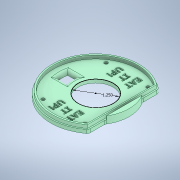
# Autodesk Inventor part: camHolderTop
Saved by Autodesk Inventor 2020 (Build 240168000, 168)
## iProperties
Created: 2020-02-08
Part Number: camHolderTop
Material: Generic
Document SubType Name: Modeling
Designer: Chris Gerth
Density: 1 g/cm^3
Appearance: Default(1)
Author: Chris Gerth
Autodesk Inventor part; units mm, degrees
ref_plane "YZ Plane" through (0, 0, 0) normal (1, 0, 0) x (0, 1, 0)
ref_plane "XZ Plane" through (0, 0, 0) normal (0, 1, 0) x (-1, 0, 0)
ref_plane "XY Plane" through (0, 0, 0) normal (0, 0, 1) x (1, 0, 0)
sketch "Sketch1" plane through (0, 0, 0) normal (0, 1, 0) x (-1, 0, 0)
  arc A0 (-25.4, -31.7246) -> (-25.4, 31.7246) centre (0, 0) ccw
  line L0 (-25.4, 31.7246) -> (-25.4, -31.7246)
  dimension "d0" = 81.28
  dimension "d21" = 25.4
  constraints: 2 end point, 2 point on circle, 1 centre point, 1 coincident, 1 vertical
  measures "d0" diameter of A0
  measures "d21" distance from line of L0 point (0, 0)
extrude "Extrusion1" add sketch "Sketch1" along normal blind 3.175
sketch "Sketch2" plane through (0, 3.175, 0) normal (0, 1, 0) x (0, 0, 1)
  circle A0 centre (0, 0) radius 40.64
  arc A1 (-31.3667, 24.003) -> (31.3667, 24.003) centre (0, 0) ccw
  arc A2 (-31.7246, 25.4) -> (31.7246, 25.4) centre (0, 0) ccw projected
  line L0 (31.7246, 25.4) -> (-31.7246, 25.4)
  line L1 (31.3667, 24.003) -> (-31.3667, 24.003)
  line L2 (30.48, 22.86) -> (-30.48, 22.86)
  arc A3 (-30.48, 22.86) -> (30.48, 22.86) centre (0, 0) ccw
  dimension "d3" = 81.28
  dimension "d5" = 78.994
  dimension "d22" = 1.397
  dimension "d23" = 1.143
  constraints: 6 end point, 4 point on circle, 3 centre point, 3 coincident, 3 horizontal
  measures "d3" diameter of A0
  measures "d5" diameter of A1
  measures "d22" distance between parallel lines of L1 L0
  measures "d23" distance between parallel lines of L1 L2
extrude "Extrusion2" add sketch "Sketch2" along normal blind 3.048 contours L1 A1
sketch "Sketch3" plane through (0, 3.175, 0) normal (0, 1, 0) x (0, 0, 1)
  circle A0 centre (0, 0) radius 15.875
  dimension "d8" = 31.75
  constraints: 1 centre point, 1 coincident
  measures "d8" diameter of A0
extrude "Extrusion3" cut sketch "Sketch3" against normal up to surface (3.175 mm away)
sketch "Sketch4" plane through (0, 3.175, 0) normal (0, 1, 0) x (0, 0, 1)
  line L0 (28.575, 19.05) -> (28.575, -19.05)
  line L1 (28.575, -19.05) -> (-28.575, -19.05)
  line L2 (-28.575, -19.05) -> (-28.575, 19.05)
  line L3 (-28.575, 19.05) -> (28.575, 19.05)
  line L4 (28.575, 19.05) -> (-28.575, -19.05) construction
  line L5 (28.575, -19.05) -> (-28.575, 19.05) construction
  circle A0 centre (-28.575, -19.05) radius 1.55
  circle A1 centre (-28.575, 19.05) radius 1.55
  circle A2 centre (28.575, 19.05) radius 1.55
  circle A3 centre (28.575, -19.05) radius 1.55
  point P0 (0, 0)
  dimension "d12" = 38.1
  dimension "d13" = 3.1
  dimension "d14" = 3.1
  dimension "d15" = 3.1
  dimension "d16" = 3.1
  dimension "d17" = 57.15
  constraints: 12 end point, 4 centre point, 4 coincident, 2 parallel, 1 perpendicular
  measures "d12" distance of L1.end L2.end
  measures "d13" diameter of A0
  measures "d14" diameter of A1
  measures "d15" diameter of A2
  measures "d16" diameter of A3
  measures "d17" distance of L0.end L1.end
extrude "Extrusion4" cut sketch "Sketch4" against normal up to surface (3.175 mm away) contours L3 A2 L0 | L0 A2 L3 | A3 L1 L0 | L0 L1 A3 | A1 L2 L3 | L3 L2 A1 | A0 L2 L1 | L1 L2 A0
sketch "Sketch5" plane through (0, 3.175, 0) normal (0, 1, 0) x (1, 0, 0)
  circle A0 centre (0, 0) radius 30.48
  line L0 (25.4, -31.7246) -> (25.4, 31.7246) projected
  line L1 (25.4, -16.8485) -> (25.4, 16.8485)
  dimension "d24" = 60.96
  constraints: 2 end point, 2 point on circle, 2 point on line, 1 centre point, 1 coincident
  measures "d24" diameter of A0
extrude "Extrusion5" add sketch "Sketch5" against normal up to surface (3.175 mm away) contours A0 L0 picked at (26.3286, -3.867)
sketch "Sketch6" plane through (0, 3.175, 0) normal (0, 1, 0) x (1, 0, 0)
  circle A0 centre (0, 0) radius 30.48
  arc A1 (25.4, -16.8485) -> (25.4, 16.8485) centre (0, 0) ccw projected
  line L0 (25.781, 16.2595) -> (25.781, -16.2595)
  line L1 (24.003, -31.3667) -> (24.003, 31.3667) projected
  point P0 (25.781, 16.2595)
  dimension "d27" = 1.778
  constraints: 2 end point, 2 point on circle, 1 centre point, 1 coincident, 1 vertical
  measures "d27" distance between parallel lines of L0 L1
extrude "Extrusion6" add sketch "Sketch6" along normal blind 3.175 contours A0 L0
fillet "Fillet1" radius 3.175 4 edges at (25.4, 1.5875, 31.7246) (25.4, 1.5875, -31.7246) (25.4, 1.5875, 16.8485) (25.4, 1.5875, -16.8485)
sketch "Sketch7" plane through (0, 3.175, 0) normal (0, 1, 0) x (1, 0, 0)
  circle A0 centre (0, 0) radius 30.2768
  circle A1 centre (0, 0) radius 22.352
  line L0 (-21.8722, -4.6064) -> (-29.9243, -4.6064)
  line L1 (-21.8866, 4.5376) -> (-29.9348, 4.5376)
  dimension "d31" = 60.5536
  dimension "d32" = 44.704
  dimension "d33" = 9.144
  constraints: 4 end point, 4 point on circle, 2 centre point, 2 coincident, 1 horizontal
  measures "d31" diameter of A0
  measures "d32" diameter of A1
  measures "d33" distance between parallel lines of L1 L0
extrude "Extrusion7" cut sketch "Sketch7" against normal up to surface (3.175 mm away) contours L1 A1 L0 A0 picked at (-24.6978, -3.5938)
fillet "Fillet2" radius 3.175 4 edges at (-22.352, 3.175, 0.0351) (-25.8983, 3.175, 4.6064) (-25.9107, 3.175, -4.5376) (-30.2768, 3.175, 0.0348)
sketch "Sketch8" plane through (0, 3.175, 0) normal (0, 1, 0) x (1, 0, 0)
  line L0 (11.4987, 33.3187) -> (11.2662, 17.0795) construction
  line L1 (11.2662, 17.0795) -> (-1.4145, 17.261) construction
  line L2 (-1.4145, 17.261) -> (-1.1821, 33.5002) construction
  line L3 (-1.1821, 33.5002) -> (11.4987, 33.3187) construction
  line L4 (11.0156, -18.9279) -> (10.7832, -35.1671) construction
  line L5 (10.7832, -35.1671) -> (-1.8976, -34.9856) construction
  line L6 (-1.8976, -34.9856) -> (-1.6651, -18.7464) construction
  line L7 (-1.6651, -18.7464) -> (11.0156, -18.9279) construction
  line L8 (6.3911, 31.4257) -> (11.4705, 31.353)
  line L9 (11.4705, 31.353) -> (11.4214, 27.92)
  line L10 (11.4214, 27.92) -> (10.4541, 27.9338)
  line L11 (10.4541, 27.9338) -> (10.4851, 30.099)
  line L12 (10.4851, 30.099) -> (9.5918, 30.1118)
  line L13 (9.5918, 30.1118) -> (9.5633, 28.1154)
  line L14 (9.5633, 28.1154) -> (8.5959, 28.1292)
  line L15 (8.5959, 28.1292) -> (8.6245, 30.1256)
  line L16 (8.6245, 30.1256) -> (7.3402, 30.144)
  line L17 (7.3402, 30.144) -> (7.3092, 27.9788)
  line L18 (7.3092, 27.9788) -> (6.3419, 27.9927)
  line L19 (6.3419, 27.9927) -> (6.3911, 31.4257)
  line L20 (6.3374, 27.6757) -> (11.3923, 25.8865)
  line L21 (11.3923, 25.8865) -> (11.3724, 24.4952)
  line L22 (11.3724, 24.4952) -> (6.2683, 22.8515)
  line L23 (6.2683, 22.8515) -> (6.2871, 24.1645)
  line L24 (6.2871, 24.1645) -> (7.329, 24.4667)
  line L25 (7.329, 24.4667) -> (7.3518, 26.0638)
  line L26 (7.3518, 26.0638) -> (6.3191, 26.3997)
  line L27 (6.3191, 26.3997) -> (6.3374, 27.6757)
  line L28 (8.255, 24.7334) -> (9.9419, 25.228)
  line L29 (9.9419, 25.228) -> (8.2699, 25.7748)
  line L30 (8.2699, 25.7748) -> (8.255, 24.7334)
  line L31 (6.2471, 21.3696) -> (10.3593, 21.3107)
  line L32 (10.3593, 21.3107) -> (10.3808, 22.8132)
  line L33 (10.3808, 22.8132) -> (11.3481, 22.7993)
  line L34 (11.3481, 22.7993) -> (11.2868, 18.5184)
  line L35 (11.2868, 18.5184) -> (10.3195, 18.5323)
  line L36 (10.3195, 18.5323) -> (10.341, 20.0347)
  line L37 (10.341, 20.0347) -> (6.2289, 20.0936)
  line L38 (6.2289, 20.0936) -> (6.2471, 21.3696)
  line L39 (-2.0492, 26.1654) -> (-2.0101, 28.8986)
  line L40 (-2.0101, 28.8986) -> (-1.1251, 28.8859)
  line L41 (-1.1251, 28.8859) -> (-1.1355, 28.1573)
  line L42 (-1.1355, 28.1573) -> (2.174, 28.11)
  line L43 (2.174, 28.11) -> (2.1844, 28.8386)
  line L44 (2.1844, 28.8386) -> (3.0694, 28.8259)
  line L45 (3.0694, 28.8259) -> (3.0303, 26.0927)
  line L46 (3.0303, 26.0927) -> (2.1453, 26.1053)
  line L47 (2.1453, 26.1053) -> (2.1557, 26.8339)
  line L48 (2.1557, 26.8339) -> (-1.1537, 26.8813)
  line L49 (-1.1537, 26.8813) -> (-1.1642, 26.1527)
  line L50 (-1.1642, 26.1527) -> (-2.0492, 26.1654)
  line L51 (-2.0753, 24.3419) -> (2.0369, 24.283)
  line L52 (2.0369, 24.283) -> (2.0584, 25.7855)
  line L53 (2.0584, 25.7855) -> (3.0257, 25.7716)
  line L54 (3.0257, 25.7716) -> (2.9644, 21.4907)
  line L55 (2.9644, 21.4907) -> (1.9971, 21.5045)
  line L56 (1.9971, 21.5045) -> (2.0186, 23.007)
  line L57 (2.0186, 23.007) -> (-2.0935, 23.0658)
  line L58 (-2.0935, 23.0658) -> (-2.0753, 24.3419)
  spline S0 degree 2 poles (-10.4805, 29.0054) (-10.4658, 30.0304) (-9.4621, 31.1194) (-8.5072, 31.1057) knots 0 0 0 1 2 2 2
  line L59 (-8.5072, 31.1057) -> (-5.2636, 31.0593)
  line L60 (-5.2636, 31.0593) -> (-5.2818, 29.7832)
  line L61 (-5.2818, 29.7832) -> (-8.4513, 29.8286)
  spline S1 degree 2 poles (-8.4513, 29.8286) (-8.9823, 29.8362) (-9.5067, 29.4444) (-9.5132, 28.9916) knots 0 0 0 1 2 2 2
  spline S2 degree 2 poles (-9.5132, 28.9916) (-9.5195, 28.5511) (-9.0273, 28.1324) (-8.4757, 28.1245) knots 0 0 0 1 2 2 2
  line L62 (-8.4757, 28.1245) -> (-5.3062, 28.0791)
  line L63 (-5.3062, 28.0791) -> (-5.3245, 26.8031)
  line L64 (-5.3245, 26.8031) -> (-8.564, 26.8494)
  spline S3 degree 2 poles (-8.564, 26.8494) (-9.5025, 26.8629) (-10.4956, 27.9516) (-10.4805, 29.0054) knots 0 0 0 1 2 2 2
  spline S4 degree 2 poles (-6.9956, 21.94) (-7.3496, 21.945) (-7.9885, 22.1806) (-8.1996, 22.3936) knots 0 0 0 1 2 2 2
  spline S5 degree 2 poles (-8.1996, 22.3936) (-8.3336, 22.5232) (-8.5514, 22.8392) (-8.6269, 23.0255) knots 0 0 0 1 2 2 2
  spline S6 degree 2 poles (-8.6269, 23.0255) (-8.7024, 23.216) (-8.7867, 23.6577) (-8.7828, 23.9294) knots 0 0 0 1 2 2 2
  line L65 (-8.7828, 23.9294) -> (-8.7733, 24.5963)
  line L66 (-8.7733, 24.5963) -> (-10.4362, 24.6201)
  line L67 (-10.4362, 24.6201) -> (-10.418, 25.8961)
  line L68 (-10.418, 25.8961) -> (-5.3385, 25.8234)
  line L69 (-5.3385, 25.8234) -> (-5.3667, 23.8517)
  spline S7 degree 2 poles (-5.3667, 23.8517) (-5.373, 23.4154) (-5.5426, 22.7797) (-5.7192, 22.5228) knots 0 0 0 1 2 2 2
  spline S8 degree 2 poles (-5.7192, 22.5228) (-5.9168, 22.2374) (-6.5552, 21.9337) (-6.9956, 21.94) knots 0 0 0 1 2 2 2
  spline S9 degree 2 poles (-7.0098, 23.2494) (-6.7917, 23.2463) (-6.48, 23.4477) (-6.4204, 23.5868) knots 0 0 0 1 2 2 2
  spline S10 degree 2 poles (-6.4204, 23.5868) (-6.3396, 23.7668) (-6.3102, 24.0958) (-6.3061, 24.3798) knots 0 0 0 1 2 2 2
  line L70 (-6.3061, 24.3798) -> (-6.3035, 24.5609)
  line L71 (-6.3035, 24.5609) -> (-7.8265, 24.5827)
  line L72 (-7.8265, 24.5827) -> (-7.8278, 24.4921)
  spline S11 degree 2 poles (-7.8278, 24.4921) (-7.8303, 24.3151) (-7.8267, 23.994) (-7.8078, 23.8743) knots 0 0 0 1 2 2 2
  spline S12 degree 2 poles (-7.8078, 23.8743) (-7.7928, 23.7711) (-7.6973, 23.5433) (-7.6364, 23.4807) knots 0 0 0 1 2 2 2
  spline S13 degree 2 poles (-7.6364, 23.4807) (-7.5148, 23.3472) (-7.2403, 23.2527) (-7.0098, 23.2494) knots 0 0 0 1 2 2 2
  line L73 (-5.4235, 19.8836) -> (-9.0356, 20.0753)
  line L74 (-9.0356, 20.0753) -> (-9.0202, 21.1538)
  line L75 (-9.0202, 21.1538) -> (-5.4041, 21.242)
  line L76 (-5.4041, 21.242) -> (-5.4235, 19.8836)
  line L77 (-10.5029, 19.9645) -> (-10.4837, 21.3065)
  line L78 (-10.4837, 21.3065) -> (-9.5822, 21.2936)
  line L79 (-9.5822, 21.2936) -> (-9.6014, 19.9516)
  line L80 (-9.6014, 19.9516) -> (-10.5029, 19.9645)
  line L81 (5.908, -20.821) -> (10.9875, -20.8937)
  line L82 (10.9875, -20.8937) -> (10.9384, -24.3266)
  line L83 (10.9384, -24.3266) -> (9.971, -24.3128)
  line L84 (9.971, -24.3128) -> (10.002, -22.1476)
  line L85 (10.002, -22.1476) -> (9.1088, -22.1349)
  line L86 (9.1088, -22.1349) -> (9.0802, -24.1312)
  line L87 (9.0802, -24.1312) -> (8.1129, -24.1174)
  line L88 (8.1129, -24.1174) -> (8.1415, -22.121)
  line L89 (8.1415, -22.121) -> (6.8572, -22.1026)
  line L90 (6.8572, -22.1026) -> (6.8262, -24.2678)
  line L91 (6.8262, -24.2678) -> (5.8589, -24.2539)
  line L92 (5.8589, -24.2539) -> (5.908, -20.821)
  line L93 (5.8543, -24.5709) -> (10.9093, -26.3601)
  line L94 (10.9093, -26.3601) -> (10.8893, -27.7514)
  line L95 (10.8893, -27.7514) -> (5.7853, -29.3952)
  line L96 (5.7853, -29.3952) -> (5.8041, -28.0821)
  line L97 (5.8041, -28.0821) -> (6.8459, -27.78)
  line L98 (6.8459, -27.78) -> (6.8688, -26.1829)
  line L99 (6.8688, -26.1829) -> (5.8361, -25.8469)
  line L100 (5.8361, -25.8469) -> (5.8543, -24.5709)
  line L101 (7.772, -27.5133) -> (9.4588, -27.0186)
  line L102 (9.4588, -27.0186) -> (7.7869, -26.4718)
  line L103 (7.7869, -26.4718) -> (7.772, -27.5133)
  line L104 (5.7641, -30.877) -> (9.8762, -30.9359)
  line L105 (9.8762, -30.9359) -> (9.8977, -29.4334)
  line L106 (9.8977, -29.4334) -> (10.8651, -29.4473)
  line L107 (10.8651, -29.4473) -> (10.8038, -33.7282)
  line L108 (10.8038, -33.7282) -> (9.8365, -33.7144)
  line L109 (9.8365, -33.7144) -> (9.858, -32.2119)
  line L110 (9.858, -32.2119) -> (5.7458, -32.1531)
  line L111 (5.7458, -32.1531) -> (5.7641, -30.877)
  line L112 (-2.5322, -26.0812) -> (-2.4931, -23.348)
  line L113 (-2.4931, -23.348) -> (-1.6081, -23.3607)
  line L114 (-1.6081, -23.3607) -> (-1.6185, -24.0893)
  line L115 (-1.6185, -24.0893) -> (1.691, -24.1366)
  line L116 (1.691, -24.1366) -> (1.7014, -23.4081)
  line L117 (1.7014, -23.4081) -> (2.5864, -23.4207)
  line L118 (2.5864, -23.4207) -> (2.5473, -26.1539)
  line L119 (2.5473, -26.1539) -> (1.6623, -26.1413)
  line L120 (1.6623, -26.1413) -> (1.6727, -25.4127)
  line L121 (1.6727, -25.4127) -> (-1.6368, -25.3653)
  line L122 (-1.6368, -25.3653) -> (-1.6472, -26.0939)
  line L123 (-1.6472, -26.0939) -> (-2.5322, -26.0812)
  line L124 (-2.5583, -27.9047) -> (1.5538, -27.9636)
  line L125 (1.5538, -27.9636) -> (1.5753, -26.4612)
  line L126 (1.5753, -26.4612) -> (2.5427, -26.475)
  line L127 (2.5427, -26.475) -> (2.4814, -30.7559)
  line L128 (2.4814, -30.7559) -> (1.5141, -30.7421)
  line L129 (1.5141, -30.7421) -> (1.5356, -29.2396)
  line L130 (1.5356, -29.2396) -> (-2.5766, -29.1808)
  line L131 (-2.5766, -29.1808) -> (-2.5583, -27.9047)
  spline S14 degree 2 poles (-10.9636, -23.2412) (-10.9489, -22.2163) (-9.9452, -21.1272) (-8.9902, -21.1409) knots 0 0 0 1 2 2 2
  line L132 (-8.9902, -21.1409) -> (-5.7466, -21.1873)
  line L133 (-5.7466, -21.1873) -> (-5.7649, -22.4634)
  line L134 (-5.7649, -22.4634) -> (-8.9344, -22.418)
  spline S15 degree 2 poles (-8.9344, -22.418) (-9.4654, -22.4104) (-9.9898, -22.8023) (-9.9962, -23.255) knots 0 0 0 1 2 2 2
  spline S16 degree 2 poles (-9.9962, -23.255) (-10.0025, -23.6955) (-9.5104, -24.1142) (-8.9588, -24.1221) knots 0 0 0 1 2 2 2
  line L135 (-8.9588, -24.1221) -> (-5.7892, -24.1675)
  line L136 (-5.7892, -24.1675) -> (-5.8075, -25.4435)
  line L137 (-5.8075, -25.4435) -> (-9.047, -25.3972)
  spline S17 degree 2 poles (-9.047, -25.3972) (-9.9855, -25.3838) (-10.9786, -24.295) (-10.9636, -23.2412) knots 0 0 0 1 2 2 2
  spline S18 degree 2 poles (-7.4787, -30.3066) (-7.8327, -30.3016) (-8.4716, -30.066) (-8.6826, -29.853) knots 0 0 0 1 2 2 2
  spline S19 degree 2 poles (-8.6826, -29.853) (-8.8166, -29.7235) (-9.0344, -29.4074) (-9.11, -29.2211) knots 0 0 0 1 2 2 2
  spline S20 degree 2 poles (-9.11, -29.2211) (-9.1855, -29.0306) (-9.2697, -28.5889) (-9.2658, -28.3172) knots 0 0 0 1 2 2 2
  line L138 (-9.2658, -28.3172) -> (-9.2563, -27.6504)
  line L139 (-9.2563, -27.6504) -> (-10.9193, -27.6266)
  line L140 (-10.9193, -27.6266) -> (-10.901, -26.3505)
  line L141 (-10.901, -26.3505) -> (-5.8215, -26.4232)
  line L142 (-5.8215, -26.4232) -> (-5.8498, -28.3949)
  spline S21 degree 2 poles (-5.8498, -28.3949) (-5.856, -28.8312) (-6.0257, -29.467) (-6.2023, -29.7238) knots 0 0 0 1 2 2 2
  spline S22 degree 2 poles (-6.2023, -29.7238) (-6.3999, -30.0092) (-7.0382, -30.313) (-7.4787, -30.3066) knots 0 0 0 1 2 2 2
  spline S23 degree 2 poles (-7.4929, -28.9972) (-7.2747, -29.0003) (-6.963, -28.7989) (-6.9034, -28.6598) knots 0 0 0 1 2 2 2
  spline S24 degree 2 poles (-6.9034, -28.6598) (-6.8226, -28.4798) (-6.7932, -28.1509) (-6.7891, -27.8668) knots 0 0 0 1 2 2 2
  line L143 (-6.7891, -27.8668) -> (-6.7865, -27.6857)
  line L144 (-6.7865, -27.6857) -> (-8.3096, -27.6639)
  line L145 (-8.3096, -27.6639) -> (-8.3109, -27.7545)
  spline S25 degree 2 poles (-8.3109, -27.7545) (-8.3134, -27.9315) (-8.3098, -28.2527) (-8.2909, -28.3723) knots 0 0 0 1 2 2 2
  spline S26 degree 2 poles (-8.2909, -28.3723) (-8.2759, -28.4755) (-8.1803, -28.7033) (-8.1195, -28.7659) knots 0 0 0 1 2 2 2
  spline S27 degree 2 poles (-8.1195, -28.7659) (-7.9979, -28.8994) (-7.7234, -28.9939) (-7.4929, -28.9972) knots 0 0 0 1 2 2 2
  line L146 (-5.9065, -32.363) -> (-9.5186, -32.1713)
  line L147 (-9.5186, -32.1713) -> (-9.5032, -31.0929)
  line L148 (-9.5032, -31.0929) -> (-5.8871, -31.0046)
  line L149 (-5.8871, -31.0046) -> (-5.9065, -32.363)
  line L150 (-10.9859, -32.2821) -> (-10.9667, -30.9402)
  line L151 (-10.9667, -30.9402) -> (-10.0652, -30.9531)
  line L152 (-10.0652, -30.9531) -> (-10.0844, -32.295)
  line L153 (-10.0844, -32.295) -> (-10.9859, -32.2821)
  point P0 (0, 0)
  constraints: 4 other
extrude "Extrusion8" cut sketch "Sketch8" against normal blind 1.016
body "Solid1"
